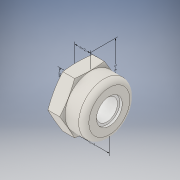
# Autodesk Inventor part: 652203A2
Saved by Autodesk Inventor 2019 (Build 230136000, 136)
## iProperties
Created: 2024-06-05
Part Number: 652203A2
Material: Generic
Catalog Web Link: www.cadenas.de
Description: DIN 985-SKM-KL-TEIL-NIEDRIG-Nuts DIN 985 (similar DIN EN ISO 10511) with Polyamide Insert, thin Version
Vendor: MAEDLER
Document SubType Name: Modeling
Designer: psAdmin
Manufacturer: MAEDLER
Mass: 0.6 g
Surface Area: 1.5508 cm^2
Volume: 0.0938207 cm^3
Density: 1 g/cm^3
Appearance: PSOLRGB-222-219-214
Category: PARTsolutions
Company: MAEDLER
Title: 652203A2
Author: Cadenas PARTsolutions
Comments: Nuts DIN 985 (similar DIN EN ISO 10511) with Polyamide Insert, thin Version
PSOL_IDENT_0: {$CADENAS_DATA/23d-libs/maedler/antriebselemente/muttern_schrauben_verbindungselemente/schrauben_mut
PSOL_IDENT_1: tern_stifte/skm_985_sichernd_nf.prj},178 {VTYP=3D},{NB=652203A2},{LINA=652203A2},{NN=DIN 985-SKM-KL-
PSOL_IDENT_2: TEIL-NIEDRIG},{DATE=26.04.2024 05:20:30},{GEOMDATE=17.02.2024 11:51:25},{VERSION=},{LINEID=630},{WBV
PSOL_IDENT_3: AR=},{WBNUMERIC=}  {NB=652203A2},{LINA=652203A2},{KT=DUMMY},{ARTNR=652203A2},{WEBSHOP=Produktdetails
PSOL_IDENT_4: / Katalogseite / Montageanleitung},{MATK=Edelstahl},{MAT=Edelstahl V2A (A2)},{AUSF=Niedrige Form},{
PSOL_IDENT_5: G=M3},{P=0.50},{H=4.0},{M=2.00},{S=6},{GEW=0.06},{TYP=2},{GG=3},{WUK=15},{DW=4.6},{SS=5.950},{ABR=0.
PSOL_IDENT_6: 28},{CTN=73181660},{DIST=0.500}
NB: 652203A2
NN: DIN 985-SKM-KL-TEIL-NIEDRIG
NT: Nuts DIN 985 (similar DIN EN ISO 10511) with Polyamide Insert, thin Version
NBSYN: $ARTNR.
LINA: 652203A2
CATALOG: MÄDLER
ARTNR: 652203A2
WEBSHOP: https://maedler.de/ShopSearch?query=652203A2
MATK: Stainless steel
MAT: Stainless Steel V2A (A2)
AUSF: Thin Version
G: M3
P: 0.5
H: 4
M: 2
S: 6
GEW: 0.06
CTN: 73181660
SUPPLIER: MAEDLER
ARTICLENO: 652203A2
BOMINFO: 652203A2
CREATOR: CADENAS GmbH
Autodesk Inventor part; units mm, degrees
ref_plane "YZ Plane" through (0, 0, 0) normal (1, 0, 0) x (0, 1, 0)
ref_plane "XZ Plane" through (0, 0, 0) normal (0, 1, 0) x (-1, 0, 0)
ref_plane "XY Plane" through (0, 0, 0) normal (0, 0, 1) x (1, 0, 0)
sketch "Sketch_1" plane through (0, 0, 0) normal (1, 0, 0) x (0, -1, 0)
  line L0 (-3, -1.7321) -> (0, -3.4641)
  line L1 (0, -3.4641) -> (3, -1.7321)
  line L2 (3, -1.7321) -> (3, 1.7321)
  line L3 (3, 1.7321) -> (0, 3.4641)
  line L4 (0, 3.4641) -> (-3, 1.7321)
  line L5 (-3, 1.7321) -> (-3, -1.7321)
  constraints: 12 end point
extrude "Extrusion1" add sketch "Sketch_1" along normal blind 2
sketch "Sketch_2" plane through (0, 0, 0) normal (0, -1, 0) x (0, 0, -1)
  line L0 (0, -50) -> (0, 50)
  line L1 (2.3, 0) -> (6, 0)
  line L2 (6, 0) -> (6, 0.9914)
  line L3 (6, 0.9914) -> (2.3, 0)
  constraints: 8 end point
revolve "Revolution1" cut sketch "Sketch_2" angle 360 about axis through (-50, 0, 0) along (-1, 0, 0)
sketch "Sketch_3" plane through (0, 0, 0) normal (0, -1, 0) x (0, 0, -1)
  line L0 (0, -50) -> (0, 50)
  line L1 (2.3, 2) -> (6, 1.0086)
  line L2 (6, 1.0086) -> (6, 2)
  line L3 (6, 2) -> (2.3, 2)
  constraints: 8 end point
revolve "Revolution2" cut sketch "Sketch_3" angle 360 about axis through (-50, 0, 0) along (-1, 0, 0)
sketch "Sketch_4" plane through (0, 0, 0) normal (0, -1, 0) x (0, 0, -1)
  line L0 (0, -200) -> (0, 200)
  line L1 (0, 4) -> (2.38, 4)
  arc A0 (2.975, 3.405) -> (2.38, 4) centre (2.38, 3.405) ccw
  line L2 (2.975, 3.405) -> (2.975, 1.7543)
  line L3 (2.975, 1.7543) -> (0, 1.7543)
  line L4 (0, 1.7543) -> (0, 4)
  constraints: 10 end point, 2 point on circle, 1 centre point
revolve "Revolution3" add sketch "Sketch_4" angle 360 about axis through (-200, 0, 0) along (-1, 0, 0)
sketch "Sketch_5" plane through (0, 0, 0) normal (0, 0, 1) x (0, -1, 0)
  line L0 (0, -200) -> (0, 200)
  line L1 (0, 2) -> (1.5, 2)
  line L2 (1.5, 2) -> (1.2295, 1.7295)
  line L3 (1.2295, 1.7295) -> (1.2295, 0.2705)
  line L4 (1.2295, 0.2705) -> (1.5, 0)
  line L5 (1.5, 0) -> (0, 0)
  line L6 (0, 0) -> (0, 2)
  constraints: 14 end point
revolve "Revolution4" cut sketch "Sketch_5" angle 360 about axis through (-200, 0, 0) along (-1, 0, 0)
thread "Thread1" size "M3x0.5" class "6H" standard "ISO Metric profile" full length
sketch "Sketch6" plane through (4, 0, 0) normal (1, 0, 0) x (0, 0, -1)
  point P0 (0, 0)
hole "Hole1" at (4, 0, 0) direction (-1, 0, 0) diameter 2.459 depth 2 counterbore diameter 3 counterbore depth 0.28
body "Solid1"
